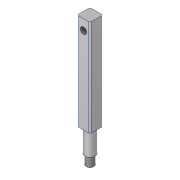
# Autodesk Inventor part: 200-60-DIFFERENTIAL-BAR-01
Saved by Autodesk Inventor 2018.2 (Build 222227000, 227)
## iProperties
Manager: feesmrt
Company: FRANC0R
Created: 2017-12-05
Part Number: 200-60-DIFFERENTIAL-BAR-01
Material: Aluminium 6061
Document SubType Name: Modeling
Designer: feesmrt
Density: 2.7 g/cm^3
Appearance: Aluminium - flach
Project: Rescue Robot
Cost Center: -
Engineer: feesmrt
Authority: feesmrt
Description: Differential Connector Bar
Stock Number: 200-60-DIFFERENTIAL-01
Author: feesmrt
Subject: Rescue Robot
Title: Differential Connector Bar
Revision Number: 1
Autodesk Inventor part; units mm, degrees
ref_plane "YZ Plane" through (0, 0, 0) normal (1, 0, 0) x (0, 1, 0)
ref_plane "XZ Plane" through (0, 0, 0) normal (0, 1, 0) x (-1, 0, 0)
ref_plane "XY Plane" through (0, 0, 0) normal (0, 0, 1) x (1, 0, 0)
sketch "Skizze3" plane through (0, 0, 0) normal (0, 0, 1) x (1, 0, 0)
  line L0 (-7, 0) -> (7, 0) construction
  line L1 (0, 7) -> (0, -7) construction
  line L2 (-5, -5) -> (5, -5)
  line L3 (5, -5) -> (5, 5)
  line L4 (5, 5) -> (-5, 5)
  line L5 (-5, 5) -> (-5, -5)
  line L6 (-5, -5) -> (5, 5) construction
  line L7 (5, -5) -> (-5, 5) construction
  point P0 (0, 0)
  dimension "d18" = 10
  constraints: 12 end point, 2 midpoint, 2 parallel, 2 perpendicular, 1 horizontal
  measures "d18" distance of L3.end L4.end
extrude "Grundkörper" add sketch "Skizze3" along normal blind 75
sketch "Skizze5" plane through (0, 0, 0) normal (1, 0, 0) x (0, 1, 0)
  line L0 (0, 5.2) -> (0, -31.2) construction
  line L1 (-5, 0) -> (5, 0) projected
  line L2 (0, 0) -> (-4, 0)
  line L3 (-4, 0) -> (-4, -18)
  line L4 (-4, -18) -> (-3, -18)
  line L5 (-3, -18) -> (-3, -26)
  line L6 (-3, -26) -> (0, -26)
  line L7 (0, -26) -> (0, 0)
  dimension "d24" = 8
  dimension "d26" = 6
  dimension "d27" = 8
  dimension "d28" = 18
  constraints: 12 end point, 3 perpendicular, 2 point on line, 1 collinear, 1 vertical
  measures "d24" diameter of L3 L0
  measures "d26" diameter of L5 L0
  measures "d27" distance of L4.end L5.end
  measures "d28" distance of L2.end L3.end
revolve "Zapfen" add sketch "Skizze5" angle 360 about axis through (0, 0, 0) along (0, 0, -1)
thread "M6_Außen" size "M6x1" class "6g" standard "ANSI Metric M Profile" full length
sketch "Skizze7" plane through (-5, 5, 0) normal (0, 1, 0) x (1, 0, 0)
  line L0 (10, -75) -> (0, -75) construction
  line L1 (5, 46.2) -> (5, -95.2) construction
  point P0 (5, 0)
  point P1 (5, -67)
  dimension "d41" = 8
  constraints: 1 point on line
  measures "d41" distance from line of L0 point (5, -67)
hole "M6_Innen" at (0, 5, 67) direction (0, -1, 0) diameter 4.917 end through all thread size "M6x1" class "6H" standard "ISO Metric profile"
chamfer "Fase_Gewinde" distance 0.5 angle 45 1 edges at (0, 3, -26)
chamfer "Fase_Allgemein" distance 1 angle 45 4 edges at (5, -5, 37.5) (5, 5, 37.5) (-5, -5, 37.5) (-5, 5, 37.5)
